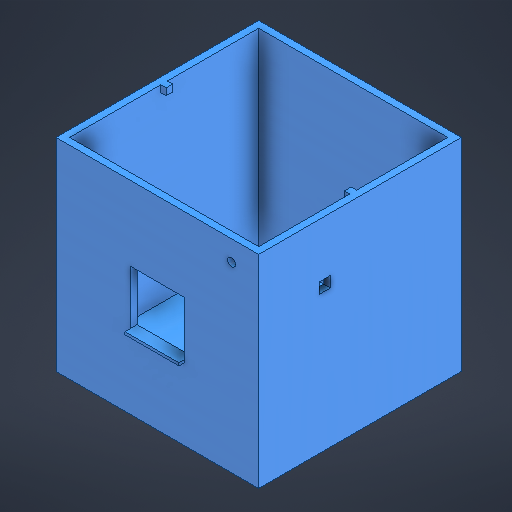
# Autodesk Inventor part: Box na elektro
Saved by Autodesk Inventor 2026.2 (Build 302298000, 298)
## iProperties
Created: 2025-09-11
Part Number: Box na elektro
Material: Všeobecné
Document SubType Name: Modeling
Designer: cerna
Density: 1 g/cm^3
Appearance: Světle modrá
Author: cerna
Autodesk Inventor part; units mm, degrees
ref_plane "YZ Plane" through (0, 0, 0) normal (1, 0, 0) x (0, 1, 0)
ref_plane "XZ Plane" through (0, 0, 0) normal (0, 1, 0) x (-1, 0, 0)
ref_plane "XY Plane" through (0, 0, 0) normal (0, 0, 1) x (1, 0, 0)
sketch "Náčrt1" plane through (0, 0, 0) normal (0, 0, 1) x (1, 0, 0)
  line L0 (0, 105) -> (0, -105) projected
  line L1 (-105, 0) -> (105, 0) projected
  line L2 (-75, 75) -> (75, 75)
  line L3 (75, 75) -> (75, -75)
  line L4 (75, -75) -> (-75, -75)
  line L5 (-75, -75) -> (-75, 75)
  point P0 (0, 0)
  dimension "d0" = 150
  dimension "d1" = 150
  constraints: 8 end point, 2 parallel, 1 horizontal, 1 perpendicular, 2 other
  measures "d0" distance of L3.end L4.end
  measures "d1" distance of L2.end L3.end
extrude "Vysunutí1" add sketch "Náčrt1" along normal blind 150
sketch "Náčrt2" plane through (-75, 75, 0) normal (0, 1, 0) x (1, 0, 0)
  line L0 (0, 0) -> (0, -150) projected
  line L1 (150, 0) -> (0, 0) projected
  line L2 (5, -145) -> (145, -145)
  line L3 (145, -145) -> (145, -5)
  line L4 (145, -5) -> (5, -5)
  line L5 (5, -5) -> (5, -145)
  point P0 (75, 0)
  dimension "d4" = 140
  dimension "d5" = 140
  dimension "d6" = 5
  dimension "d7" = 5
  constraints: 8 end point, 2 parallel, 1 horizontal, 1 perpendicular
  measures "d4" distance of L4.end L3.end
  measures "d5" distance of L3.end L2.end
  measures "d6" distance between parallel lines of L1 L4
  measures "d7" distance between parallel lines of L0 L5
extrude "Vysunutí2" cut sketch "Náčrt2" against normal blind 140
sketch "Náčrt3" plane through (0, 0, 150) normal (0, 0, 1) x (1, 0, 0)
  line L0 (-20, 20) -> (20, 20)
  line L1 (20, 20) -> (20, -20)
  line L2 (20, -20) -> (-20, -20)
  line L3 (-20, -20) -> (-20, 20)
  line L4 (0, 105) -> (0, -105) projected
  line L5 (-105, 0) -> (105, 0) projected
  line L6 (-75, -75) -> (75, -75) projected
  circle A0 centre (55, 60) radius 3
  line L7 (75, -75) -> (75, 75) projected
  line L8 (75, 75) -> (-75, 75) projected
  point P0 (0, 0)
  dimension "d10" = 40
  dimension "d11" = 40
  dimension "d12" = 55
  dimension "d13" = 6
  dimension "d14" = 20
  dimension "d15" = 15
  constraints: 8 end point, 2 parallel, 1 centre point, 1 horizontal, 1 perpendicular, 1 other
  measures "d10" distance of L1.end L2.end
  measures "d11" distance of L0.end L1.end
  measures "d12" distance between parallel lines of L6 L2
  measures "d13" diameter of A0
  measures "d14" distance from line of L7 A0.centre
  measures "d15" distance from line of L8 A0.centre
extrude "Vysunutí3" cut sketch "Náčrt3" against normal blind 10 contours L0 L4 L5 L3 | L0 L1 L5 L4 | L5 L4 L2 L3 | L5 L1 L2 L4 | A0
sketch "Náčrt36" plane through (75, -75, 0) normal (1, 0, 0) x (0, 0, -1)
  line L0 (-105, 110) -> (-97, 110)
  line L1 (-97, 110) -> (-97, 102)
  line L2 (-97, 102) -> (-105, 102)
  line L3 (-105, 102) -> (-105, 110)
  line L4 (0, 0) -> (0, 150) projected
  line L5 (0, 150) -> (-150, 150) projected
  line L6 (-150, 0) -> (-150, 150) projected
  line L7 (0, 0) -> (-150, 0) projected
  point P0 (0, 75)
  dimension "d188" = 8
  dimension "d189" = 8
  dimension "d190" = 40
  dimension "d191" = 45
  constraints: 8 end point, 2 parallel, 1 horizontal, 1 perpendicular
  measures "d188" distance of L0.start L0.end
  measures "d189" distance of L0.end L1.end
  measures "d190" distance between parallel lines of L5 L0
  measures "d191" distance between parallel lines of L6 L3
extrude "Vysunutí28" cut sketch "Náčrt36" against normal blind 10 contours L0 L1 L2 L3
sketch "Náčrt37" plane through (0, 0, 150) normal (0, 0, 1) x (1, 0, 0)
  line L0 (-20, -20) -> (-20, 20) projected
  line L1 (-20, -20) -> (20, -20)
  line L2 (20, -20) -> (20, -22)
  line L3 (20, -22) -> (-20, -22)
  line L4 (-20, -22) -> (-20, -20)
  point P0 (0, 0)
  dimension "d194" = 2
  dimension "d195" = 40
  constraints: 8 end point, 2 parallel, 1 horizontal, 1 perpendicular
  measures "d194" distance of L1.end L2.end
  measures "d195" distance of L2.end L3.end
extrude "Vysunutí29" add sketch "Náčrt37" along normal blind 4
sketch "Náčrt38" plane through (-70, 75, 145) normal (1, 0, 0) x (0, 0, -1)
  line L0 (0, 0) -> (140, 0) projected
  line L1 (0, 0) -> (0, -140) projected
  line L2 (0, -140) -> (140, -140) projected
  line L3 (140, 0) -> (140, -140) projected
  line L4 (67.5, 0) -> (72.5, 0)
  line L5 (72.5, 0) -> (72.5, -5)
  line L6 (72.5, -5) -> (67.5, -5)
  line L7 (67.5, -5) -> (67.5, 0)
  point P0 (145, -75)
  dimension "d198" = 5
  dimension "d199" = 5
  dimension "d200" = 67.5
  constraints: 8 end point, 2 parallel, 1 horizontal, 1 perpendicular, 1 point on line
  measures "d198" distance of L5.end L6.end
  measures "d199" distance of L4.end L5.end
  measures "d200" distance between parallel lines of L7 L1
extrude "Vysunutí30" add sketch "Náčrt38" along normal blind 4 contours L0 L5 L6 L7
sketch "Náčrt39" plane through (70, 75, 5) normal (-1, 0, 0) x (0, 0, 1)
  line L0 (92, -48) -> (92, -40) projected
  line L1 (92, -40) -> (100, -40) projected
  line L2 (100, -40) -> (100, -48) projected
  line L3 (100, -48) -> (92, -48) projected
  line L4 (0, 0) -> (140, 0) projected
  line L5 (0, 0) -> (0, -140) projected
  line L6 (0, -140) -> (140, -140) projected
  line L7 (140, 0) -> (140, -140) projected
  line L8 (67.5, 0) -> (72.5, 0)
  line L9 (72.5, 0) -> (72.5, -5)
  line L10 (72.5, -5) -> (67.5, -5)
  line L11 (67.5, -5) -> (67.5, 0)
  point P0 (-5, -75)
  point P1 (72.5, 0)
  dimension "d203" = 5
  dimension "d204" = 5
  dimension "d205" = 67.5
  constraints: 8 end point, 2 parallel, 1 horizontal, 1 perpendicular, 1 point on line
  measures "d203" distance of L8.end L9.end
  measures "d204" distance of L9.end L10.end
  measures "d205" distance between parallel lines of L5 L11
extrude "Vysunutí31" add sketch "Náčrt39" along normal blind 4 contours L4 L9 L10 L11
sketch "Náčrt41" plane through (0, 0, 0) normal (0, 0, -1) x (-1, 0, 0)
  line L0 (75, -75) -> (-75, -75) projected
  line L1 (75, 75) -> (75, -75) projected
  line L2 (-75, 75) -> (75, 75) projected
  line L3 (-75, -75) -> (-75, 75) projected
  line L4 (-7, -45) -> (7, -45)
  line L5 (7, -45) -> (7, -55)
  line L6 (7, -55) -> (-7, -55)
  line L7 (-7, -55) -> (-7, -45)
  line L8 (0, -105) -> (0, 105) projected
  point P0 (0, 0)
  dimension "d209" = 14
  dimension "d210" = 10
  dimension "d211" = 20
  constraints: 8 end point, 2 parallel, 1 horizontal, 1 perpendicular, 1 other
  measures "d209" distance of L5.end L6.end
  measures "d210" distance of L4.end L5.end
  measures "d211" distance between parallel lines of L0 L6
extrude "Vysunutí32" cut sketch "Náčrt41" against normal blind 10 contours L8 L4 L5 L6 | L6 L7 L4 L8
